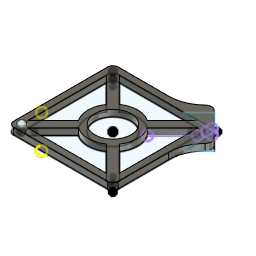
Qube (Autodesk Fusion 360 design; units mm, degrees)
Autodesk Fusion 360 part; units mm, degrees
sketch "스케치1" plane through (0, 0, 0) normal (0, 0, 1) x (1, 0, 0)
  line L0 (-36, 40) -> (36, 40)
  line L1 (40, 36) -> (40, -36)
  line L2 (36, -40) -> (-36, -40)
  line L3 (-40, -36) -> (-40, 36)
  line L4 (-30, 35) -> (30, 35)
  line L5 (35, 30) -> (35, -30)
  line L6 (30, -35) -> (-30, -35)
  line L7 (-35, -30) -> (-35, 30)
  arc A0 (-36, 40) -> (-40, 36) centre (-36, 36) ccw
  arc A1 (40, 36) -> (36, 40) centre (36, 36) ccw
  arc A2 (36, -40) -> (40, -36) centre (36, -36) ccw
  arc A3 (-40, -36) -> (-36, -40) centre (-36, -36) ccw
  arc A4 (-35, -30) -> (-30, -35) centre (-30, -30) ccw
  arc A5 (30, -35) -> (35, -30) centre (30, -30) ccw
  arc A6 (35, 30) -> (30, 35) centre (30, 30) ccw
  arc A7 (-30, 35) -> (-35, 30) centre (-30, 30) ccw
  line L8 (-35, -30) -> (-15.7004, -10.7004)
  line L9 (10.7004, 15.7004) -> (30, 35)
  line L10 (-30, -35) -> (-10.7004, -15.7004)
  line L11 (15.7004, 10.7004) -> (35, 30)
  line L12 (-35, 30) -> (-15.7004, 10.7004)
  line L13 (10.7004, -15.7004) -> (30, -35)
  line L14 (-30, 35) -> (-10.7004, 15.7004)
  line L15 (15.7004, -10.7004) -> (35, -30)
  circle A8 centre (0, 0) radius 14
  arc A9 (-10.7004, -15.7004) -> (10.7004, -15.7004) centre (0, 0) ccw
  arc A10 (15.7004, -10.7004) -> (15.7004, 10.7004) centre (0, 0) ccw
  arc A11 (10.7004, 15.7004) -> (-10.7004, 15.7004) centre (0, 0) ccw
  arc A12 (-15.7004, 10.7004) -> (-15.7004, -10.7004) centre (0, 0) ccw
  point P0 (-40, 40)
  point P1 (40, 40)
  point P2 (40, -40)
  point P3 (-35, 35)
  point P4 (35, -35)
  point P5 (-35, -35)
  dimension "d1" = 80
  dimension "d2" = 80
  dimension "d3" = 40
  dimension "d4" = 40
  dimension "d5" = 70
  dimension "d6" = 70
  dimension "d7" = 5
  dimension "d8" = 5
  dimension "d9" = 4
  dimension "d10" = 38
  dimension "d11" = 5
  dimension "d12" = 28
  constraint horizontal L0
  constraint vertical L1
  constraint horizontal L2
  constraint vertical L3
  constraint horizontal L4
  constraint vertical L5
  constraint horizontal L6
  constraint vertical L7
  constraint coincident P0 L0
  constraint coincident P0 L3
  constraint tangent L0 A0
  constraint tangent L3 A0
  constraint coincident P1 L0
  constraint coincident P1 L1
  constraint tangent L0 A1
  constraint tangent L1 A1
  constraint equal A0 A1
  constraint coincident P2 L1
  constraint coincident P2 L2
  constraint tangent L1 A2
  constraint tangent L2 A2
  constraint equal A0 A2
  constraint tangent L2 A3
  constraint tangent L3 A3
  constraint equal A0 A3
  constraint coincident A8.centre A9.centre
  constraint coincident P5 L6
  constraint coincident P5 L7
  constraint tangent L6 A4
  constraint tangent L7 A4
  constraint coincident P4 L5
  constraint coincident P4 L6
  constraint tangent L5 A5
  constraint tangent L6 A5
  constraint equal A4 A5
  constraint tangent L4 A6
  constraint tangent L5 A6
  constraint equal A4 A6
  constraint coincident P3 L4
  constraint coincident P3 L7
  constraint tangent L4 A7
  constraint tangent L7 A7
  constraint equal A4 A7
  constraint coincident L9.start A9
  constraint collinear L8 L9
  constraint coincident L11.start A9
  constraint collinear L10 L11
  constraint coincident L12.end A9
  constraint collinear L12 L13
  constraint coincident L14.end A9
  constraint coincident L15.start A9
  constraint collinear L14 L15
  constraint concentric A9 A10
  constraint concentric A10 A11
  constraint concentric A11 A12
  measures "d1" distance of P1 P2
  measures "d2" distance of P0 P1
  measures "d3" distance of A8.centre L1
  measures "d4" distance of A8.centre L2
  measures "d5" distance of P3 P5
  measures "d6" distance of P4 P5
  measures "d7" distance of L0 L4
  measures "d8" distance of L1 L5
  measures "d9" radius of A0
  measures "d10" diameter of A9
  measures "d11" radius of A4
  measures "d12" diameter of A8
extrude "돌출1" add sketch "스케치1" along normal blind 5 contours L0 L1 L2 L3 A0 A1 A2 A3 | A4 A5 A6 A7 L8 L9 L10 L11 L12 L13 L14 L15 A9 A10 A11 A12
sketch "스케치2" plane through (0, 0, 5) normal (0, 0, 1) x (-1, 0, 0)
  circle A0 centre (35, 35) radius 1.7
  dimension "d15" = 3.4
  measures "d15" diameter of A0
extrude "돌출2" cut sketch "스케치2" against normal through all
sketch "스케치9" plane through (0, 0, 0) normal (0, 0, -1) x (1, 0, 0)
  line L0 (15.7004, -10.7004) -> (35, -30)
  arc A0 (36, -40) -> (40, -36) centre (36, -36) ccw construction
  line L1 (51.5725, -26.0844) -> (40, -14.5118) construction
  line L2 (40, -14.5118) -> (51.5725, -26.0844)
  line L3 (38.8284, -38.8284) -> (51.5725, -26.0844)
  line L4 (40, -14.5118) -> (38.8284, -38.8284)
  line L5 (38.8284, -38.8284) -> (26.0844, -51.5725)
  line L6 (14.5118, -40) -> (38.8284, -38.8284)
  line L7 (14.5118, -40) -> (26.0844, -51.5725)
  point P0 (-14.5118, 40)
  point P1 (-40, 14.5118)
  constraint midpoint A0 L3.start
  constraint tangent A0 L3
extrude "돌출6" add sketch "스케치9" against normal blind 5
sketch "스케치10" plane through (38.8284, 38.8284, 0) normal (0.707107, 0.707107, 0) x (-0.707107, 0.707107, 0)
  circle A0 centre (-9.7, 2.5) radius 1.7
  line L0 (0, 0) -> (0, -7)
  circle A1 centre (9.7, 2.5) radius 1.7
  dimension "d46" = 3.4
  dimension "d47" = 9.7
  constraint symmetric A0 L0 A1
  measures "d46" diameter of A0
  measures "d47" horizontal distance of A0.centre L0.start
extrude "돌출7" cut sketch "스케치10" against normal blind 2
sketch "스케치11" plane through (37.4142, 37.4142, 0) normal (0.707107, 0.707107, 0) x (-0.707107, 0.707107, 0)
  circle A0 centre (-9.7, 2.5) radius 1.25
  circle A1 centre (9.7, 2.5) radius 1.25
  point P0 (-9.7, 2.5)
  point P1 (9.7, 2.5)
  dimension "d50" = 2.5
  dimension "d51" = 2.5
  constraint coincident P0 A0.centre
  constraint coincident P1 A1.centre
  measures "d50" diameter of A0
  measures "d51" diameter of A1
extrude "돌출8" cut sketch "스케치11" against normal blind 2
fillet "모깎기1" radius 5 2 edges at (26.0844, 51.5725, 2.5) (51.5725, 26.0844, 2.5)
fillet "모깎기2" radius 28.5 2 edges at (40, 14.5118, 2.5) (14.5118, 40, 2.5)
